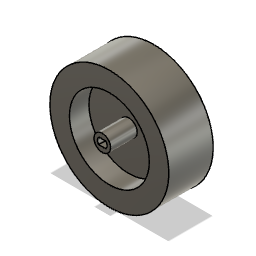
rueda_simple v2 (Autodesk Fusion 360 design; units mm, degrees)
Autodesk Fusion 360 part; units mm, degrees
sketch "Sketch1" plane through (0, 0, 0) normal (0, 0, 1) x (1, 0, 0)
  circle A0 centre (0, 0) radius 33.5
  dimension "d1" = 67
  constraint coincident A0.centre origin
  measures "d1" diameter of A0
extrude "Extrude1" add sketch "Sketch1" against normal blind 25
sketch "Sketch2" plane through (0, 0, 0) normal (0, 0, 1) x (1, 0, 0)
  circle A0 centre (0, 0) radius 4.7
  circle A1 centre (0, 0) radius 2.75
  line L0 (2.75, 1.875) -> (-2.75, 1.875)
  line L1 (-2.75, 1.875) -> (-2.75, -1.875)
  line L2 (-2.75, -1.875) -> (2.75, -1.875)
  line L3 (2.75, -1.875) -> (2.75, 1.875)
  line L4 (2.75, 1.875) -> (-2.75, -1.875) construction
  line L5 (-2.75, 1.875) -> (2.75, -1.875) construction
  dimension "d4" = 9.4
  dimension "d7" = 5.5
  dimension "d8" = 3.75
  constraint coincident A0.centre A1.centre
  constraint horizontal L0
  constraint perpendicular L0 L1
  constraint parallel L0 L2
  constraint parallel L1 L3
  constraint coincident L4 A0.centre
  constraint coincident L5 A0.centre
  constraint tangent A1 L3
  measures "d4" diameter of A0
  measures "d7" diameter of A1
  measures "d8" distance of L0.start L2.end
extrude "Extrude2" add sketch "Sketch2" along normal blind 4 contours A0 | A1 L0 L2 | A1 L2 L3 | A1 L0 L3 | A1 L0 | A1 L2 | A1 L0 L1 | A1 L1 L2
extrude "Extrude3" cut sketch "Sketch2" along normal blind 7 and the other way blind 20 contours A1 L0 L2
sketch "Sketch3" plane through (0, 0, 0) normal (0, 0, 1) x (1, 0, 0)
  circle A0 centre (0, 0) radius 4.7
  circle A1 centre (0, 0) radius 33.5
  circle A2 centre (0, 0) radius 22.5
  line L0 (-2.0117, 1.875) -> (2.0117, 1.875)
  arc A3 (2.0117, -1.875) -> (2.0117, 1.875) centre (0, 0) ccw
  line L1 (2.0117, -1.875) -> (-2.0117, -1.875)
  arc A4 (-2.0117, 1.875) -> (-2.0117, -1.875) centre (0, 0) ccw
  circle A5 centre (0, 0) radius 4.7
  dimension "d13" = 45
  constraint coincident A0.centre A1.centre
  measures "d13" diameter of A2
extrude "Extrude4" cut sketch "Sketch3" against normal blind 11 contours A2
